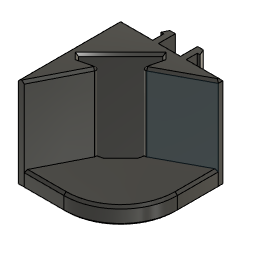
Led CLip v1 (Autodesk Fusion 360 design; units mm, degrees)
Autodesk Fusion 360 part; units mm, degrees
sketch "Sketch1" plane through (0, 0, 0) normal (0, 0, 1) x (1, 0, 0)
  line L0 (18, -0.8) -> (18, 0)
  line L1 (9, -0.8) -> (9, 0) construction
  line L2 (7.05, 0) -> (7.05, 2.5936)
  line L3 (7.05, 2.5936) -> (6.05, 2.5936)
  line L4 (6.05, 2.5936) -> (5.55, 1.55)
  line L5 (5.55, 1.55) -> (6.05, 1.55)
  line L6 (6.05, 1.55) -> (6.05, 0)
  line L7 (11.95, 1.55) -> (11.95, 0)
  line L8 (10.95, 0) -> (10.95, 2.5936)
  line L9 (10.95, 2.5936) -> (11.95, 2.5936)
  line L10 (11.95, 2.5936) -> (12.45, 1.55)
  line L11 (12.45, 1.55) -> (11.95, 1.55)
  line L12 (6.05, 0) -> (0, 0)
  line L13 (18, 0) -> (11.95, 0)
  line L14 (10.95, 0) -> (7.05, 0)
  line L15 (0, 0) -> (0, -0.8)
  line L16 (0, -0.8) -> (18, -0.8) construction
  line L17 (9, -0.8) -> (9, -0.7834) construction
  line L18 (5.3123, -5.3123) -> (9.2034, -9.2034) construction
  line L19 (5.209, -9.8072) -> (1.0346, -18)
  line L20 (2.3071, -9.7317) -> (4.7045, -9.165)
  line L21 (1.6, -9.0246) -> (2.3071, -9.7317)
  line L22 (5.3123, -5.3123) -> (1.6, -9.0246)
  line L23 (18, 0) -> (18, -0.8)
  arc A0 (5.209, -9.8072) -> (4.7045, -9.165) centre (4.808, -9.6029) ccw
  line L24 (0, -18) -> (0, 0)
  arc A1 (9.165, -4.7045) -> (9.8162, -5.2043) centre (9.6029, -4.808) ccw
  line L25 (9.7317, -2.3071) -> (9.165, -4.7045)
  line L26 (9.0246, -1.6) -> (9.7317, -2.3071)
  line L27 (5.3123, -5.3123) -> (9.0246, -1.6)
  line L28 (0, -18) -> (1.0346, -18)
  line L29 (9.8162, -5.2043) -> (18, -0.8)
  dimension "d13" = 1
  dimension "d14" = 115.6
  dimension "d15" = 1.55
  dimension "d16" = 0.5
  dimension "d24" = 2.95
  dimension "d25" = 18
  dimension "d26" = 0.8
  dimension "d30" = 0.45
  dimension "d45" = 121.7
  dimension "d49" = 5.25
  dimension "d50" = 1
  dimension "d52" = 45
  dimension "d53" = 1.6
  dimension "d55" = 18
  dimension "d56" = 2.6774
  dimension "d57" = 72
  dimension "d59" = 1.6
  constraint vertical L0
  constraint horizontal L13
  constraint perpendicular L2 L13
  constraint perpendicular L2 L3
  constraint perpendicular L2 L5
  constraint coincident L6.end L13
  constraint perpendicular L6 L13
  constraint coincident L3.end L6
  constraint symmetric L1 L2.start L8.start
  constraint symmetric L1 L2.end L8.end
  constraint symmetric L1 L3.end L9.end
  constraint symmetric L1 L4.end L10.end
  constraint symmetric L1 L5.end L7.start
  constraint symmetric L1 L6.end L7.end
  constraint collinear L12 L13
  constraint coincident L1.end L13
  constraint collinear L13 L14
  constraint coincident L12.end L15.start
  constraint perpendicular L12 L15
  constraint horizontal L16
  constraint midpoint L1.start L16
  constraint collinear L1 L17
  constraint tangent L20 A0
  constraint tangent L19 A0
  constraint vertical L24
  constraint symmetric L18 L20.start L25.start
  constraint symmetric L18 L21.start L26.start
  constraint symmetric L18 L20.end A1.start
  constraint symmetric L18 A0 A1
  constraint symmetric L18 L22.start L27.start
  constraint horizontal L28
  constraint tangent A1 L29
  constraint perpendicular L18 L22
  constraint perpendicular L21 L22
  measures "d13" distance of L2.end L3.end
  measures "d14" angle of L3 L4
  measures "d15" distance of L5.end L6.end
  measures "d16" distance of L4.end L6
  measures "d24" distance of L1 L6
  measures "d25" distance of L0.start L15.end
  measures "d26" distance of L12.end L15.end
  measures "d30" radius of A0
  measures "d45" angle of L20 L21
  measures "d49" distance of L21.start L18.start
  measures "d50" distance of L20.start L21.start
  measures "d52" angle of L16 L22
  measures "d53" distance of L14 L26.start
  measures "d55" distance of L24.start L12.end
  measures "d56" distance of L22 A0.centre
  measures "d57" angle of L18 L19
  measures "d59" horizontal distance of L12.end L21.start
extrude "Extrude1" add sketch "Sketch1" along normal blind 13.5
sketch "Sketch5" plane through (0, 0, 0) normal (0, 0, -1) x (1, 0, 0)
  line L0 (9.0246, 1.6) -> (1.6, 9.0246)
  line L1 (1.6, 9.0246) -> (2.3071, 9.7317)
  line L2 (2.3071, 9.7317) -> (4.7045, 9.165)
  arc A0 (4.7045, 9.165) -> (5.209, 9.8072) centre (4.808, 9.6029) ccw
  line L3 (5.209, 9.8072) -> (1.0346, 18)
  line L4 (1.0346, 18) -> (0, 18)
  line L5 (0, 18) -> (0, 0)
  line L6 (0, 0) -> (6.05, 0)
  line L7 (6.05, 0) -> (6.05, -1.55)
  line L8 (6.05, -1.55) -> (5.55, -1.55)
  line L9 (5.55, -1.55) -> (6.05, -2.5936)
  line L10 (6.05, -2.5936) -> (7.05, -2.5936)
  line L11 (7.05, -2.5936) -> (7.05, 0)
  line L12 (7.05, 0) -> (10.95, 0)
  line L13 (10.95, 0) -> (10.95, -2.5936)
  line L14 (10.95, -2.5936) -> (11.95, -2.5936)
  line L15 (11.95, -2.5936) -> (12.45, -1.55)
  line L16 (12.45, -1.55) -> (11.95, -1.55)
  line L17 (11.95, -1.55) -> (11.95, 0)
  line L18 (11.95, 0) -> (18, 0)
  line L19 (18, 0) -> (18, 0.8)
  line L20 (18, 0.8) -> (9.8162, 5.2043)
  arc A1 (9.8162, 5.2043) -> (9.165, 4.7045) centre (9.6029, 4.808) ccw
  line L21 (9.165, 4.7045) -> (9.7317, 2.3071)
  line L22 (9.7317, 2.3071) -> (9.0246, 1.6)
  line L23 (2.3071, 9.7317) -> (1.6, 9.0246)
  line L24 (1.6, 9.0246) -> (9.0246, 1.6)
  line L25 (9.0246, 1.6) -> (9.7317, 2.3071)
  line L26 (9.7317, 2.3071) -> (8.8561, 6.0111)
  line L27 (8.8561, 6.0111) -> (6.0111, 8.8561)
  line L28 (6.0111, 8.8561) -> (2.3071, 9.7317)
  line L29 (18, 0.8) -> (18, 8)
  line L30 (8, 18) -> (1.0346, 18)
  arc A2 (18, 8) -> (8, 18) centre (8, 8) ccw
  dimension "d62" = 3
  dimension "d63" = 10
  constraint coincident L1.end L2.start
  constraint coincident L0.end L1.start
  constraint coincident L0.start L22.end
  constraint coincident L21.end L22.start
  constraint parallel L21 L26
  constraint perpendicular L22 L27
  constraint collinear L2 L28
  constraint coincident L19.end L20.start
  constraint perpendicular L4 L29
  constraint coincident L3.end L4.start
  constraint horizontal L30
  constraint tangent L29 A2
  constraint tangent L30 A2
  measures "d62" distance of L0.start L27
  measures "d63" radius of A2
extrude "Extrude5" add sketch "Sketch5" along normal blind 3 contours L0 L1 L2 A0 L3 L4 L5 L6 L7 L8 L9 L10 L11 L12 L13 L14 L15 L16 L17 L18 L19 L20 A1 L21 L22 L23 L24 L25 L26 L28 | A0 L3 L20 A1 L26 L27 L28 L29 L30 A2
chamfer "Chamfer5" distance 0.4 angle 45 3 edges at (18, -4.4, 0) (15.0711, -15.0711, 0) (4.5173, -18, 0)
chamfer "Chamfer6" distance 0.4 angle 45 15 edges at (18, -0.4, -3) (18, -4.4, -3) (15.0711, -15.0711, -3) (4.5173, -18, -3) (0.5173, -18, -3) (14.975, 0, -3) (3.025, 0, -3) (9, 0, -3) (0, -9, -3) (5.3123, -5.3123, -3) (7.4336, -7.4336, -3) (4.1591, -9.2939, -3) (1.9536, -9.3782, -3) (9.3782, -1.9536, -3) (9.2939, -4.1591, -3)
chamfer "Chamfer7" distance 0.4 angle 45 8 edges at (9.4484, -3.5058, 13.5) (9.329, -5.165, 13.5) (13.9081, -3.0021, 13.5) (5.3123, -5.3123, 13.5) (3.1218, -13.9036, 13.5) (5.1619, -9.325, 13.5) (3.5058, -9.4484, 13.5) (0, -9, 13.5)
chamfer "Chamfer8" distance 0.4 angle 45 2 edges at (9.403, -1.9784, 13.5) (1.9784, -9.403, 13.5)
chamfer "Chamfer9" distance 0.4 angle 45 3 edges at (7.4336, -7.4336, 0) (5.3578, -9.0106, 0) (9.0106, -5.3578, 0)
chamfer "Chamfer10" distance 0.4 angle 45 4 edges at (14.975, 0, 13.5) (9, 0, 13.5) (3.225, 0, 13.5) (18, -0.1729, 13.5)
sketch "Sketch6" plane through (4.3763, -8.1319, 0) normal (0.473902, -0.880578, 0) x (0.880578, 0.473902, 0)
  line L0 (15.4713, 13.1) -> (6.1776, 13.1)
  line L1 (6.1776, 13.1) -> (6.1776, 0)
  line L2 (6.1776, 0) -> (15.017, 0)
  line L3 (15.017, 0) -> (15.4713, -0.4)
  line L4 (15.4713, -0.4) -> (15.4713, 13.1)
named bodies: "Light Bar Clip - Misumi"
